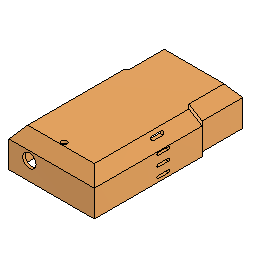
cover (Autodesk Fusion 360 design; units mm, degrees)
Autodesk Fusion 360 part; units mm, degrees
ref_plane "WorkPlane1" through (0.2066, 15.7648, 8.9) normal (0, 0, 1) x (1, 0, 0)
sketch "Sketch2" plane through (0, 0, 8.9) normal (0, 0, 1) x (1, 0, 0)
  line L0 (29.7, -34.1) -> (29.7, -44.1)
  line L1 (29.7, -44.1) -> (-29.7, -44.1)
  line L2 (-29.7, -44.1) -> (-29.7, -34.1)
  line L3 (-29.7, -34.1) -> (-29.7, 33.9793)
  line L4 (26.4759, 36.7) -> (29.7, 33.4759)
  line L5 (29.7, 33.4759) -> (29.7, -34.1)
  line L6 (26.4759, 36.7) -> (26.4759, 65.8)
  line L7 (26.4759, 65.8) -> (-27.7, 65.8)
  line L8 (-27.7, 36.7) -> (-29.7, 33.9793)
  line L9 (-28, 36.7984) -> (-28, 66.1)
  line L10 (-27.7, 41.6) -> (-27.7, 61.3)
  line L11 (-29.7, -34.1) -> (-29.7, 33.9793)
  line L12 (-29.7, -44.1) -> (-29.7, -34.1)
  line L13 (29.7, -44.1) -> (-29.7, -44.1)
  line L14 (29.7, -34.1) -> (29.7, -44.1)
  line L15 (29.7, 33.4759) -> (29.7, -34.1)
  line L16 (26.4759, 36.7) -> (29.7, 33.4759)
  line L17 (26.4759, 36.7) -> (26.4759, 65.8)
  line L18 (26.4759, 65.8) -> (-27.7, 65.8)
  line L19 (-30, -34.1) -> (-30, 34.0777)
  line L20 (-30, -44.4) -> (-30, -34.1)
  line L21 (30, -44.4) -> (-30, -44.4)
  line L22 (30, -34.1) -> (30, -44.4)
  line L23 (30, 33.6001) -> (30, -34.1)
  line L24 (26.7759, 36.8243) -> (30, 33.6001)
  line L25 (26.7759, 36.8243) -> (26.7759, 66.1)
  line L26 (26.7759, 66.1) -> (-28, 66.1)
  line L27 (-30, 34.0777) -> (-28, 36.7984)
  line L28 (-27.7, 36.7) -> (-29.7, 33.9793)
  line L29 (-27.7, 65.8) -> (-27.7, 36.7)
  line L30 (32, -46.4) -> (-32, -46.4)
  line L31 (-32, -46.4) -> (-32, -34.1)
  line L32 (-32, -34.1) -> (-32, 34.7337)
  line L33 (-32, 34.7337) -> (-30, 37.4544)
  line L34 (-30, 37.4544) -> (-30, 68.1)
  line L35 (28.7759, 68.1) -> (-30, 68.1)
  line L36 (28.7759, 37.6527) -> (28.7759, 68.1)
  line L37 (28.7759, 37.6527) -> (32, 34.4286)
  line L38 (32, 34.4286) -> (32, -34.1)
  line L39 (32, -34.1) -> (32, -46.4)
  dimension "d197" = 0.3
  dimension "d241" = 0.3
  dimension "d245" = -2
  constraint vertical L9
  constraint coincident L8.start L28.start
  constraint coincident L3.end L8.end
  constraint equal L27 L28
  constraint coincident L7.end L18.end
  constraint collinear L4 L16
  constraint collinear L6 L17
  constraint collinear L7 L18
  measures "d197" distance of L9 L10
  measures "d241" distance of L27 L28
extrude "Extrude8" add sketch "Sketch2" against normal blind 29 contours L0 L1 L2 L3 L4 L5 L6 L7 L8 L10 L11 L12 L13 L14 L15 L16 L17 L18 L28 L29 | L9 L19 L20 L21 L22 L23 L24 L25 L26 L27 | L30 L31 L32 L33 L34 L35 L36 L37 L38 L39
chamfer "Chamfer3" distance 7 distance2 9 1 faces at (-10.6667, 11.6874, 8.9)
shell "Shell2" thickness 2 removed faces 1 at (-10.6667, 7.5874, -20.1)
sketch "Sketch6" plane through (-32, 0, 0) normal (-1, 0, 0) x (0, 1, 0)
  line L0 (12.55, -46.4) -> (12.55, 35.1337)
  line L1 (12.55, 35.1337) -> (-7.45, 35.1337)
  line L2 (-7.45, 35.1337) -> (-7.45, -46.4)
  line L3 (-7.45, -46.4) -> (12.55, -46.4)
  line L4 (1.55, 23.4141) -> (9.05, 23.4141)
  arc A0 (9.05, 23.4141) -> (9.05, 25.4141) centre (9.05, 24.4141) ccw
  line L5 (9.05, 25.4141) -> (1.55, 25.4141)
  arc A1 (1.55, 25.4141) -> (1.55, 23.4141) centre (1.55, 24.4141) ccw
  line L6 (1.55, 24.4141) -> (9.05, 24.4141) construction
  line L7 (9.05, 17.8601) -> (1.55, 17.8601)
  arc A2 (1.55, 17.8601) -> (1.55, 15.8601) centre (1.55, 16.8601) ccw
  arc A3 (9.05, 15.8601) -> (9.05, 17.8601) centre (9.05, 16.8601) ccw
  line L8 (1.55, 15.8601) -> (9.05, 15.8601)
  line L9 (9.05, 10.3061) -> (1.55, 10.3061)
  arc A4 (1.55, 10.3061) -> (1.55, 8.3061) centre (1.55, 9.3061) ccw
  arc A5 (9.05, 8.3061) -> (9.05, 10.3061) centre (9.05, 9.3061) ccw
  line L10 (1.55, 8.3061) -> (9.05, 8.3061)
  line L11 (9.05, 2.7521) -> (1.55, 2.7521)
  arc A6 (1.55, 2.7521) -> (1.55, 0.7521) centre (1.55, 1.7521) ccw
  arc A7 (9.05, 0.7521) -> (9.05, 2.7521) centre (9.05, 1.7521) ccw
  line L12 (1.55, 0.7521) -> (9.05, 0.7521)
  line L13 (9.05, -4.8019) -> (1.55, -4.8019)
  arc A8 (1.55, -4.8019) -> (1.55, -6.8019) centre (1.55, -5.8019) ccw
  arc A9 (9.05, -6.8019) -> (9.05, -4.8019) centre (9.05, -5.8019) ccw
  line L14 (1.55, -6.8019) -> (9.05, -6.8019)
  line L15 (-46.4, 0.1) -> (34.7337, 0.1)
  line L16 (34.7337, 0.1) -> (34.7337, 20.1)
  line L17 (34.7337, 20.1) -> (-46.4, 20.1)
  line L18 (-46.4, 20.1) -> (-46.4, 0.1)
  point P0 (2.174, 24.4141)
  dimension "d187" = 2
  dimension "d200" = 0
  dimension "d201" = -30.216
  dimension "d232" = 9
  dimension "d233" = 3.5
  constraint tangent L4 A0
  constraint tangent A0 L5
  constraint parallel L4 L5
  constraint tangent L5 A1
  constraint tangent L4 A1
  constraint coincident A1.centre L6.start
  constraint coincident A0.centre L6.end
  constraint horizontal A1.centre P0
  constraint horizontal L6
  measures "d187" distance of L4 L5
  measures "d232" distance of L2 A1.centre
  measures "d233" distance of L0 A0.centre
extrude "Extrude9" cut sketch "Sketch6" against normal blind 64 contours L4 A0 L5 A1 | L7 A2 A3 L8 | L9 A4 A5 L10 | L11 A6 A7 L12 | L13 A8 A9 L14
sketch "Sketch7" plane through (0, -46.4, 0) normal (0, -1, 0) x (1, 0, 0)
  line L0 (-32, -12.55) -> (32, -12.55)
  line L1 (32, -12.55) -> (32, 7.45)
  line L2 (32, 7.45) -> (-32, 7.45)
  line L3 (-32, 7.45) -> (-32, -12.55)
  circle A0 centre (-16.7045, -6.5) radius 3.25
  circle A1 centre (-16.7045, -6.5) radius 5
  dimension "d258" = 10
  constraint concentric A0 A1
  measures "d258" diameter of A1
extrude "Extrude11" cut sketch "Sketch7" against normal blind 2 contours A0 | A1
sketch "Sketch8" plane through (0, 0, 8.9) normal (0, 0, 1) x (-1, 0, 0)
  line L0 (21.7759, 34.7532) -> (21.7759, 61.1)
  line L1 (21.7759, 61.1) -> (-23, 61.1)
  line L2 (-23, 61.1) -> (-23, 35.1584)
  line L3 (-23, 35.1584) -> (-25, 32.4376)
  line L4 (-25, 32.4376) -> (-25, -39.4)
  line L5 (-25, -39.4) -> (25, -39.4)
  line L6 (25, -39.4) -> (25, 31.5291)
  line L7 (25, 31.5291) -> (21.7759, 34.7532)
  circle A0 centre (0, 36.95) radius 1.9
  circle A1 centre (0, 36.95) radius 2.15
  dimension "d261" = 4.3
  constraint concentric A0 A1
  measures "d261" diameter of A1
extrude "Extrude12" cut sketch "Sketch8" against normal blind 2 contours A0 | A1
named bodies: "ezp32_cover"
